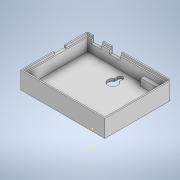
# Autodesk Inventor part: Shell 3 bottom
Saved by Autodesk Inventor 2022 (Build 260153000, 153)
## iProperties
Created: 2021-10-12
Part Number: Shell 3 bottom
Material: Generic
Document SubType Name: Modeling
Designer: Elisabeth
Density: 1 g/cm^3
Appearance: Default
Author: Elisabeth
Autodesk Inventor part; units mm, degrees
ref_plane "YZ Plane" through (0, 0, 0) normal (1, 0, 0) x (0, 1, 0)
ref_plane "XZ Plane" through (0, 0, 0) normal (0, 1, 0) x (-1, 0, 0)
ref_plane "XY Plane" through (0, 0, 0) normal (0, 0, 1) x (1, 0, 0)
sketch "Sketch1" plane through (0, 0, 0) normal (0, 1, 0) x (-1, 0, 0)
  point P0 (0, 0)
sketch "Sketch2" plane through (0, 0, 0) normal (0, 1, 0) x (-1, 0, 0)
  line L0 (70, -12) -> (70, -66)
  line L1 (70, -66) -> (2, -66)
  line L2 (70, -12) -> (2, -12)
  line L3 (2, -66) -> (2, -12)
  point P0 (0, 0)
  point P1 (2, 0)
  dimension "d151" = 68
  dimension "d152" = 54
  constraints: 8 end point, 1 perpendicular, 1 point on line
  measures "d151" distance between parallel lines of L0 L3
  measures "d152" distance between parallel lines of L1 L2
extrude "Extrusion1" add sketch "Sketch2" along normal blind 14
sketch "Sketch3" plane through (0, 14, 0) normal (0, 1, 0) x (1, 0, 0)
  point P0 (0, 0)
sketch "Sketch4" plane through (0, 14, 0) normal (0, 1, 0) x (1, 0, 0)
  line L0 (-2, 66) -> (-70, 66) projected
  line L1 (-30.4814, 66) -> (-28.4814, 66)
  line L2 (-28.4814, 66) -> (-28.4814, 64)
  line L3 (-70, 66) -> (-70, 12) projected
  line L4 (-70, 37.8423) -> (-70, 39.8423)
  line L5 (-70, 39.8423) -> (-68, 39.8423)
  line L6 (-68, 64) -> (-68, 14)
  line L7 (-68, 64) -> (-4, 64)
  line L8 (-68, 14) -> (-4, 14)
  line L9 (-4, 14) -> (-4, 64)
  line L10 (-70, 12) -> (-2, 12) projected
  line L11 (-2, 12) -> (-2, 66) projected
  point P0 (-2, 64)
  point P1 (-68, 12)
  dimension "d6" = 2
  dimension "d8" = 2
  dimension "d102" = 2
  dimension "d104" = 2
  dimension "d153" = 2
  dimension "d154" = 2
  constraints: 16 end point, 4 point on line, 3 perpendicular, 1 horizontal, 1 parallel
  measures "d6" distance of L1.end L2.end
  measures "d8" distance of L4.end L5.end
  measures "d102" distance between parallel lines of L6 L3
  measures "d104" distance between parallel lines of L7 L0
  measures "d153" distance between parallel lines of L8 L10
  measures "d154" distance between parallel lines of L11 L9
extrude "Extrusion2" cut sketch "Sketch4" against normal blind 12 contours L7 L9 L8 L6
sketch "Sketch10" plane through (0, 2, 0) normal (0, 1, 0) x (1, 0, 0)
  line L0 (-48, 14) -> (-48, 17)
  line L1 (-48, 14) -> (-63, 14)
  line L2 (-63, 14) -> (-63, 17)
  line L3 (-63, 17) -> (-48, 17)
  line L4 (-48, 17) -> (-48, 14)
  line L5 (-22, 64) -> (-7, 64)
  line L6 (-7, 64) -> (-7, 61)
  line L7 (-7, 61) -> (-22, 61)
  line L8 (-22, 61) -> (-22, 64)
  line L9 (-68, 64) -> (-4, 64) projected
  line L10 (-63, 14) -> (-48, 14)
  line L11 (-4, 14) -> (-68, 14) projected
  point P0 (-68, 2)
  point P1 (-2, 64)
  dimension "d55" = 3
  dimension "d56" = 15
  dimension "d60" = 15
  dimension "d108" = 3
  dimension "d155" = 0
  constraints: 20 end point, 4 parallel, 2 horizontal, 2 perpendicular
  measures "d55" distance of L0.start L0.end
  measures "d56" distance of L2.end L3.end
  measures "d60" distance of L6.end L7.end
  measures "d108" distance between parallel lines of L5 L7
  measures "d155" distance between parallel lines of L11 L1
extrude "Extrusion5" add sketch "Sketch10" along normal blind 6
sketch "Sketch12" plane through (0, 0, 0) normal (0, -1, 0) x (1, 0, 0)
  line L0 (0, 0) -> (0, -66) projected
  arc A0 (-34, -55.9641) -> (-34, -49.0359) centre (-36, -52.5) ccw
  arc A1 (-38, -58.6498) -> (-34, -58.6498) centre (-36, -58.6498) ccw
  line L1 (-34, -58.6498) -> (-34, -55.9641)
  line L2 (-38, -58.6498) -> (-38, -55.9641)
  arc A2 (-34, -49.0359) -> (-38, -55.9641) centre (-36, -52.5) ccw
  line L3 (-2, -12) -> (-2, -66) projected
  line L4 (-2, -66) -> (-70, -66) projected
  line L5 (-2, -66) -> (-70, -66)
  line L6 (-36, -66) -> (-36, -12)
  line L7 (-70, -66) -> (-70, -12) projected
  line L8 (-70, -66) -> (-70, -12)
  line L9 (-70, -39) -> (-2, -39)
  line L10 (-36, -39) -> (-36, -66)
  line L11 (-36, -52.5) -> (-2, -52.5)
  arc A3 (-39, -58.6498) -> (-33, -58.6498) centre (-36, -58.6498) ccw
  line L12 (-39, -58.6498) -> (-39, -56.5)
  arc A4 (-33.5, -48.1699) -> (-39, -56.5) centre (-36, -52.5) ccw
  arc A5 (-33, -56.5) -> (-33.5, -48.1699) centre (-36, -52.5) ccw
  line L13 (-33, -56.5) -> (-33, -58.6498)
  dimension "d156" = 34
  dimension "d157" = 1
  constraints: 20 end point, 12 point on circle, 6 centre point, 5 midpoint, 3 vertical, 2 collinear, 2 point on line, 2 tangent, 1 perpendicular, 5 other
  measures "d156" distance between parallel lines of L6 L3
  measures "d157" radial gap between concentric circles of A1 A3
extrude "Extrusion7" cut sketch "Sketch12" against normal blind 5 contours L1 A1 L6 L11 A0 | L11 L6 A2 A0 | L6 A1 L2 A2
sketch "Sketch13" plane through (0, 14, 0) normal (0, 1, 0) x (1, 0, 0)
  line L0 (-70, 66) -> (-70, 12) projected
  line L1 (-69, 65) -> (-69, 13)
  line L2 (-2, 66) -> (-70, 66) projected
  line L3 (-68, 64) -> (-4, 64)
  line L4 (-2, 64) -> (-2, 12)
  line L5 (-68, 14) -> (-68, 64)
  line L6 (-4, 14) -> (-68, 14) projected
  line L7 (-68, 14) -> (-4, 14)
  line L8 (-7, 64) -> (-4, 64) projected
  line L9 (-4, 14) -> (-4, 64)
  line L10 (-70, 12) -> (-2, 12) projected
  line L11 (-68, 13) -> (-69, 13)
  line L12 (-68, 13) -> (-3, 13)
  line L13 (-2, 12) -> (-2, 66) projected
  line L14 (-4, 13) -> (-3, 13)
  line L15 (-3, 13) -> (-3, 64)
  line L16 (-3, 64) -> (-3, 65)
  line L17 (-3, 65) -> (-69, 65)
  dimension "d96" = 1
  dimension "d99" = 1
  constraints: 24 end point, 5 perpendicular, 4 point on line, 2 collinear, 1 horizontal, 1 parallel
  measures "d96" distance between parallel lines of L0 L1
  measures "d99" distance between parallel lines of L1 L5
extrude "Extrusion8" cut sketch "Sketch13" against normal blind 2 contours L17 L16 L15 L12 L11 L1 | L3 L9 L6 L5
sketch "Sketch15" plane through (-70, 0, -66) normal (-1, 0, 0) x (0, 0, 1)
  line L0 (62.4242, 8) -> (52.7396, 8)
  line L1 (0, 0) -> (66, 0) projected
  line L2 (0, 14) -> (54, 14) projected
  line L3 (0, 0) -> (0, 14) projected
  line L4 (18.77, 12) -> (27.77, 12)
  line L5 (27.77, 12) -> (27.77, 17)
  line L6 (27.77, 17) -> (18.77, 17)
  line L7 (18.77, 17) -> (18.77, 12)
  point P0 (66, 14)
  dimension "d118" = 8
  dimension "d140" = 27.77
  dimension "d141" = 9
  dimension "d143" = 5
  dimension "d150" = 4
  constraints: 10 end point, 2 horizontal, 2 parallel, 1 perpendicular
  measures "d118" distance between parallel lines of L1 L0
  measures "d140" distance between parallel lines of L3 L5
  measures "d141" distance of L4.start L4.end
  measures "d143" distance between parallel lines of L4 L6
  measures "d150" distance between parallel lines of L0 L4
extrude "Extrusion9" cut sketch "Sketch15" against normal blind 10
sketch "Sketch16" plane through (-2, 0, -66) normal (0, 0, -1) x (-1, 0, 0)
  line L0 (39.4, 14) -> (47.9, 14)
  line L1 (47.9, 14) -> (47.9, 9)
  line L2 (47.9, 9) -> (39.4, 9)
  line L3 (39.4, 9) -> (39.4, 14)
  line L4 (54.5, 14) -> (63, 14)
  line L5 (63, 14) -> (63, 9)
  line L6 (63, 9) -> (54.5, 9)
  line L7 (54.5, 9) -> (54.5, 14)
  line L8 (20, 8) -> (5, 8) projected
  line L9 (68, 0) -> (68, 14) projected
  point P0 (-2, 0)
  dimension "d127" = 8.5
  dimension "d128" = 8.5
  dimension "d131" = 28.6
  dimension "d132" = 13.5
  dimension "d148" = 5
  dimension "d149" = 6
  constraints: 16 end point, 4 parallel, 2 horizontal, 2 perpendicular, 2 point on line
  measures "d127" distance of L1.end L2.end
  measures "d128" distance of L5.end L6.end
  measures "d131" distance between parallel lines of L3 L9
  measures "d132" distance between parallel lines of L7 L9
  measures "d148" distance of L0.end L1.end
  measures "d149" distance between parallel lines of L0 L8
extrude "Extrusion10" cut sketch "Sketch16" against normal blind 10
fillet "Fillet7" radius 2 1 edges at (-2, 7, -66)
fillet "Fillet8" radius 2 1 edges at (-70, 7, -66)
body "Solid1"
